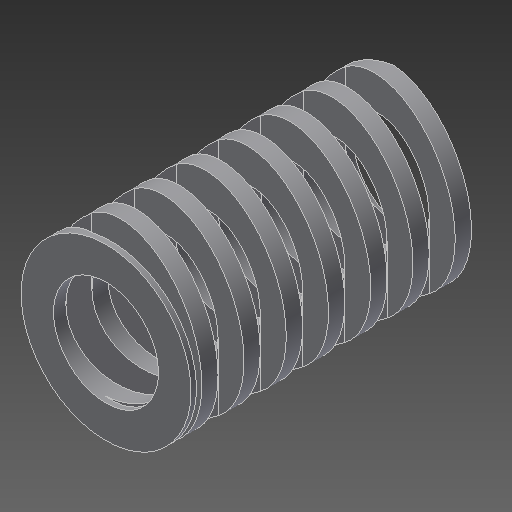
# Autodesk Inventor part: SWU17-30
Saved by Autodesk Inventor 2021.1 (Build 251245010, 245A)
## iProperties
Created: 2010-03-11
Part Number: SWU17-30
Catalog Web Link: www.cadenas.de
Document SubType Name: Modeling
Density: 1 g/cm^3
Material: MISUMI
Appearance: 既定
Category: PARTsolutions
NB: SWU17-30
NN: SWU
NT: Coil Springs - Super High Deflection - SWU
NBSYN: $PN.
LINA: SWU17-30
PN: SWU17-30
TYPE: SWU
MAT: Alloy Steel
D: 17.0
DD: 10.5
L: 30
L1: 20,25,30,35,40,45,50,55,60,65,70,75,80,90,100,110,120,125,150,175
LO: 8.17 {0.83}
LL: 9.00
F: 18.0
LO1: 147.1 {15.0}
X: 3.250
D1: 1.625
H1: 4.224
ANGLE: 5.000
KT: DUMMY
PSOL_IDENT_0: {\\10.0.0.149\dplatte\cadenas\23d-libs\misumi\metric\29_springs\swu.prj},156 {VTYP=3D},{NB=SWU17-30}
PSOL_IDENT_1: ,{LINA=SWU17-30},{NN=SWU},{DATE=18.02.2010 11:50:29},{GEOMDATE=18.02.2010 11:50:00},{VERSION=},{LINE
PSOL_IDENT_2: ID=40},{LINESUBID=-1},{WBVAR=L}  {NB=SWU17-30},{LINA=SWU17-30},{KT=DUMMY},{PN=SWU17-30},{TYPE=SWU},{
PSOL_IDENT_3: MAT=Alloy Steel},{D=17.0},{DD=10.5},{L=30},{L1=20,25,30,35,40,45,50,55,60,65,70,75,80,90,100,110,120
PSOL_IDENT_4: ,125,150,175},{LO=8.17 \{0.83\}},{LL=9.00},{F=18.0},{LO1=147.1 \{15.0\}},{X=3.25},{D1=1.625},{H1=4.2
PSOL_IDENT_5: 24},{ANGLE=5.000}
Title: コイルスプリング
Comments: Coil Springs - Super High Deflection - SWU
Autodesk Inventor part; units mm, degrees
ref_plane "YZ Plane" through (0, 0, 0) normal (1, 0, 0) x (0, 1, 0)
ref_plane "XZ Plane" through (0, 0, 0) normal (0, 1, 0) x (-1, 0, 0)
ref_plane "XY Plane" through (0, 0, 0) normal (0, 0, 1) x (1, 0, 0)
sketch "Sketch_1" plane through (0, 0, 0) normal (0, 0, 1) x (1, 0, 0)
  circle A0 centre (0, 0) radius 8.5
  circle A1 centre (0, 0) radius 5.25
  constraints: 2 centre point
extrude "Extrusion1" add sketch "Sketch_1" along normal blind 30
sketch "Sketch_2" plane through (0, 0, 0) normal (0, 1, 0) x (-1, 0, 0)
  line L0 (70.217, 56.4456) -> (8.5, 216.2365)
  line L1 (8.5, 216.2365) -> (8.5, 215.2652)
  line L2 (8.5, 215.2652) -> (5.25, 214.6115)
  line L3 (5.25, 214.6115) -> (-8.5, 217.3772)
  line L4 (-8.5, 217.3772) -> (-8.5, 214.7782)
  line L5 (-8.5, 214.7782) -> (5.25, 212.0125)
  line L6 (5.25, 212.0125) -> (8.5, 212.6662)
  line L7 (8.5, 212.6662) -> (8.5, 211.0412)
  line L8 (8.5, 211.0412) -> (5.25, 210.3875)
  line L9 (5.25, 210.3875) -> (-8.5, 213.1532)
  line L10 (-8.5, 213.1532) -> (-8.5, 210.5542)
  line L11 (-8.5, 210.5542) -> (5.25, 207.7885)
  line L12 (5.25, 207.7885) -> (8.5, 208.4422)
  line L13 (8.5, 208.4422) -> (8.5, 206.8172)
  line L14 (8.5, 206.8172) -> (5.25, 206.1635)
  line L15 (5.25, 206.1635) -> (-8.5, 208.9292)
  line L16 (-8.5, 208.9292) -> (-8.5, 206.3302)
  line L17 (-8.5, 206.3302) -> (5.25, 203.5645)
  line L18 (5.25, 203.5645) -> (8.5, 204.2182)
  line L19 (8.5, 204.2182) -> (8.5, 202.5932)
  line L20 (8.5, 202.5932) -> (5.25, 201.9395)
  line L21 (5.25, 201.9395) -> (-8.5, 204.7052)
  line L22 (-8.5, 204.7052) -> (-8.5, 202.1062)
  line L23 (-8.5, 202.1062) -> (5.25, 199.3405)
  line L24 (5.25, 199.3405) -> (8.5, 199.9942)
  line L25 (8.5, 199.9942) -> (8.5, 198.3692)
  line L26 (8.5, 198.3692) -> (5.25, 197.7155)
  line L27 (5.25, 197.7155) -> (-8.5, 200.4812)
  line L28 (-8.5, 200.4812) -> (-8.5, 197.8822)
  line L29 (-8.5, 197.8822) -> (5.25, 195.1165)
  line L30 (5.25, 195.1165) -> (8.5, 195.7702)
  line L31 (8.5, 195.7702) -> (8.5, 194.1452)
  line L32 (8.5, 194.1452) -> (5.25, 193.4915)
  line L33 (5.25, 193.4915) -> (-8.5, 196.2572)
  line L34 (-8.5, 196.2572) -> (-8.5, 193.6582)
  line L35 (-8.5, 193.6582) -> (5.25, 190.8925)
  line L36 (5.25, 190.8925) -> (8.5, 191.5462)
  line L37 (8.5, 191.5462) -> (8.5, 189.9212)
  line L38 (8.5, 189.9212) -> (5.25, 189.2675)
  line L39 (5.25, 189.2675) -> (-8.5, 192.0332)
  line L40 (-8.5, 192.0332) -> (-8.5, 189.4342)
  line L41 (-8.5, 189.4342) -> (5.25, 186.6685)
  line L42 (5.25, 186.6685) -> (8.5, 187.3222)
  line L43 (8.5, 187.3222) -> (8.5, 185.6972)
  line L44 (8.5, 185.6972) -> (5.25, 185.0435)
  line L45 (5.25, 185.0435) -> (-8.5, 187.8092)
  line L46 (-8.5, 187.8092) -> (-8.5, 185.2102)
  line L47 (-8.5, 185.2102) -> (5.25, 182.4445)
  line L48 (5.25, 182.4445) -> (8.5, 183.0982)
  line L49 (8.5, 183.0982) -> (8.5, 181.4732)
  line L50 (8.5, 181.4732) -> (5.25, 180.8195)
  line L51 (5.25, 180.8195) -> (-8.5, 183.5852)
  line L52 (-8.5, 183.5852) -> (-8.5, 180.9862)
  line L53 (-8.5, 180.9862) -> (5.25, 178.2205)
  line L54 (5.25, 178.2205) -> (8.5, 178.8742)
  line L55 (8.5, 178.8742) -> (8.5, 177.2492)
  line L56 (8.5, 177.2492) -> (5.25, 176.5955)
  line L57 (5.25, 176.5955) -> (-8.5, 179.3612)
  line L58 (-8.5, 179.3612) -> (-8.5, 176.7622)
  line L59 (-8.5, 176.7622) -> (5.25, 173.9965)
  line L60 (5.25, 173.9965) -> (8.5, 174.6502)
  line L61 (8.5, 174.6502) -> (8.5, 173.0252)
  line L62 (8.5, 173.0252) -> (5.25, 172.3715)
  line L63 (5.25, 172.3715) -> (-8.5, 175.1372)
  line L64 (-8.5, 175.1372) -> (-8.5, 172.5382)
  line L65 (-8.5, 172.5382) -> (5.25, 169.7725)
  line L66 (5.25, 169.7725) -> (8.5, 170.4262)
  line L67 (8.5, 170.4262) -> (8.5, 168.8012)
  line L68 (8.5, 168.8012) -> (5.25, 168.1475)
  line L69 (5.25, 168.1475) -> (-8.5, 170.9132)
  line L70 (-8.5, 170.9132) -> (-8.5, 168.3142)
  line L71 (-8.5, 168.3142) -> (5.25, 165.5485)
  line L72 (5.25, 165.5485) -> (8.5, 166.2022)
  line L73 (8.5, 166.2022) -> (8.5, 164.5772)
  line L74 (8.5, 164.5772) -> (5.25, 163.9235)
  line L75 (5.25, 163.9235) -> (-8.5, 166.6892)
  line L76 (-8.5, 166.6892) -> (-8.5, 164.0902)
  line L77 (-8.5, 164.0902) -> (5.25, 161.3245)
  line L78 (5.25, 161.3245) -> (8.5, 161.9782)
  line L79 (8.5, 161.9782) -> (8.5, 160.3532)
  line L80 (8.5, 160.3532) -> (5.25, 159.6995)
  line L81 (5.25, 159.6995) -> (-8.5, 162.4652)
  line L82 (-8.5, 162.4652) -> (-8.5, 159.8662)
  line L83 (-8.5, 159.8662) -> (5.25, 157.1005)
  line L84 (5.25, 157.1005) -> (8.5, 157.7542)
  line L85 (8.5, 157.7542) -> (8.5, 156.1292)
  line L86 (8.5, 156.1292) -> (5.25, 155.4755)
  line L87 (5.25, 155.4755) -> (-8.5, 158.2412)
  line L88 (-8.5, 158.2412) -> (-8.5, 155.6422)
  line L89 (-8.5, 155.6422) -> (5.25, 152.8765)
  line L90 (5.25, 152.8765) -> (8.5, 153.5302)
  line L91 (8.5, 153.5302) -> (8.5, 151.9052)
  line L92 (8.5, 151.9052) -> (5.25, 151.2515)
  line L93 (5.25, 151.2515) -> (-8.5, 154.0172)
  line L94 (-8.5, 154.0172) -> (-8.5, 151.4182)
  line L95 (-8.5, 151.4182) -> (5.25, 148.6525)
  line L96 (5.25, 148.6525) -> (8.5, 149.3062)
  line L97 (8.5, 149.3062) -> (8.5, 147.6812)
  line L98 (8.5, 147.6812) -> (5.25, 147.0275)
  line L99 (5.25, 147.0275) -> (-8.5, 149.7932)
  line L100 (-8.5, 149.7932) -> (-8.5, 147.1942)
  line L101 (-8.5, 147.1942) -> (5.25, 144.4285)
  line L102 (5.25, 144.4285) -> (8.5, 145.0822)
  line L103 (8.5, 145.0822) -> (8.5, 143.4572)
  line L104 (8.5, 143.4572) -> (5.25, 142.8035)
  line L105 (5.25, 142.8035) -> (-8.5, 145.5692)
  line L106 (-8.5, 145.5692) -> (-8.5, 142.9702)
  line L107 (-8.5, 142.9702) -> (5.25, 140.2045)
  line L108 (5.25, 140.2045) -> (8.5, 140.8582)
  line L109 (8.5, 140.8582) -> (8.5, 139.2332)
  line L110 (8.5, 139.2332) -> (5.25, 138.5795)
  line L111 (5.25, 138.5795) -> (-8.5, 141.3452)
  line L112 (-8.5, 141.3452) -> (-8.5, 138.7462)
  line L113 (-8.5, 138.7462) -> (5.25, 135.9805)
  line L114 (5.25, 135.9805) -> (8.5, 136.6342)
  line L115 (8.5, 136.6342) -> (8.5, 135.0092)
  line L116 (8.5, 135.0092) -> (5.25, 134.3555)
  line L117 (5.25, 134.3555) -> (-8.5, 137.1212)
  line L118 (-8.5, 137.1212) -> (-8.5, 134.5222)
  line L119 (-8.5, 134.5222) -> (5.25, 131.7565)
  line L120 (5.25, 131.7565) -> (8.5, 132.4102)
  line L121 (8.5, 132.4102) -> (8.5, 130.7852)
  line L122 (8.5, 130.7852) -> (5.25, 130.1315)
  line L123 (5.25, 130.1315) -> (-8.5, 132.8972)
  line L124 (-8.5, 132.8972) -> (-8.5, 130.2982)
  line L125 (-8.5, 130.2982) -> (5.25, 127.5325)
  line L126 (5.25, 127.5325) -> (8.5, 128.1862)
  line L127 (8.5, 128.1862) -> (8.5, 126.5612)
  line L128 (8.5, 126.5612) -> (5.25, 125.9075)
  line L129 (5.25, 125.9075) -> (-8.5, 128.6732)
  line L130 (-8.5, 128.6732) -> (-8.5, 126.0742)
  line L131 (-8.5, 126.0742) -> (5.25, 123.3085)
  line L132 (5.25, 123.3085) -> (8.5, 123.9622)
  line L133 (8.5, 123.9622) -> (8.5, 122.3372)
  line L134 (8.5, 122.3372) -> (5.25, 121.6835)
  line L135 (5.25, 121.6835) -> (-8.5, 124.4492)
  line L136 (-8.5, 124.4492) -> (-8.5, 121.8502)
  line L137 (-8.5, 121.8502) -> (5.25, 119.0845)
  line L138 (5.25, 119.0845) -> (8.5, 119.7382)
  line L139 (8.5, 119.7382) -> (8.5, 118.1132)
  line L140 (8.5, 118.1132) -> (5.25, 117.4595)
  line L141 (5.25, 117.4595) -> (-8.5, 120.2252)
  line L142 (-8.5, 120.2252) -> (-8.5, 117.6262)
  line L143 (-8.5, 117.6262) -> (5.25, 114.8605)
  line L144 (5.25, 114.8605) -> (8.5, 115.5142)
  line L145 (8.5, 115.5142) -> (8.5, 113.8892)
  line L146 (8.5, 113.8892) -> (5.25, 113.2355)
  line L147 (5.25, 113.2355) -> (-8.5, 116.0012)
  line L148 (-8.5, 116.0012) -> (-8.5, 113.4022)
  line L149 (-8.5, 113.4022) -> (5.25, 110.6365)
  line L150 (5.25, 110.6365) -> (8.5, 111.2902)
  line L151 (8.5, 111.2902) -> (8.5, 109.6652)
  line L152 (8.5, 109.6652) -> (5.25, 109.0115)
  line L153 (5.25, 109.0115) -> (-8.5, 111.7772)
  line L154 (-8.5, 111.7772) -> (-8.5, 109.1782)
  line L155 (-8.5, 109.1782) -> (5.25, 106.4125)
  line L156 (5.25, 106.4125) -> (8.5, 107.0662)
  line L157 (8.5, 107.0662) -> (8.5, 105.4412)
  line L158 (8.5, 105.4412) -> (5.25, 104.7875)
  line L159 (5.25, 104.7875) -> (-8.5, 107.5532)
  line L160 (-8.5, 107.5532) -> (-8.5, 104.9542)
  line L161 (-8.5, 104.9542) -> (5.25, 102.1885)
  line L162 (5.25, 102.1885) -> (8.5, 102.8422)
  line L163 (8.5, 102.8422) -> (8.5, 101.2172)
  line L164 (8.5, 101.2172) -> (5.25, 100.5635)
  line L165 (5.25, 100.5635) -> (-8.5, 103.3292)
  line L166 (-8.5, 103.3292) -> (-8.5, 100.7302)
  line L167 (-8.5, 100.7302) -> (5.25, 97.9645)
  line L168 (5.25, 97.9645) -> (8.5, 98.6182)
  line L169 (8.5, 98.6182) -> (8.5, 96.9932)
  line L170 (8.5, 96.9932) -> (5.25, 96.3395)
  line L171 (5.25, 96.3395) -> (-8.5, 99.1052)
  line L172 (-8.5, 99.1052) -> (-8.5, 96.5062)
  line L173 (-8.5, 96.5062) -> (5.25, 93.7405)
  line L174 (5.25, 93.7405) -> (8.5, 94.3942)
  line L175 (8.5, 94.3942) -> (8.5, 92.7692)
  line L176 (8.5, 92.7692) -> (5.25, 92.1155)
  line L177 (5.25, 92.1155) -> (-8.5, 94.8812)
  line L178 (-8.5, 94.8812) -> (-8.5, 92.2822)
  line L179 (-8.5, 92.2822) -> (5.25, 89.5165)
  line L180 (5.25, 89.5165) -> (8.5, 90.1702)
  line L181 (8.5, 90.1702) -> (8.5, 88.5452)
  line L182 (8.5, 88.5452) -> (5.25, 87.8915)
  line L183 (5.25, 87.8915) -> (-8.5, 90.6572)
  line L184 (-8.5, 90.6572) -> (-8.5, 88.0582)
  line L185 (-8.5, 88.0582) -> (5.25, 85.2925)
  line L186 (5.25, 85.2925) -> (8.5, 85.9462)
  line L187 (8.5, 85.9462) -> (8.5, 84.3212)
  line L188 (8.5, 84.3212) -> (5.25, 83.6675)
  line L189 (5.25, 83.6675) -> (-8.5, 86.4332)
  line L190 (-8.5, 86.4332) -> (-8.5, 83.8342)
  line L191 (-8.5, 83.8342) -> (5.25, 81.0685)
  line L192 (5.25, 81.0685) -> (8.5, 81.7222)
  line L193 (8.5, 81.7222) -> (8.5, 80.0972)
  line L194 (8.5, 80.0972) -> (5.25, 79.4435)
  line L195 (5.25, 79.4435) -> (-8.5, 82.2092)
  line L196 (-8.5, 82.2092) -> (-8.5, 79.6102)
  line L197 (-8.5, 79.6102) -> (5.25, 76.8445)
  line L198 (5.25, 76.8445) -> (8.5, 77.4982)
  line L199 (8.5, 77.4982) -> (8.5, 75.8732)
  line L200 (8.5, 75.8732) -> (5.25, 75.2195)
  line L201 (5.25, 75.2195) -> (-8.5, 77.9852)
  line L202 (-8.5, 77.9852) -> (-8.5, 75.3862)
  line L203 (-8.5, 75.3862) -> (5.25, 72.6205)
  line L204 (5.25, 72.6205) -> (8.5, 73.2742)
  line L205 (8.5, 73.2742) -> (8.5, 71.6492)
  line L206 (8.5, 71.6492) -> (5.25, 70.9955)
  line L207 (5.25, 70.9955) -> (-8.5, 73.7612)
  line L208 (-8.5, 73.7612) -> (-8.5, 71.1622)
  line L209 (-8.5, 71.1622) -> (5.25, 68.3965)
  line L210 (5.25, 68.3965) -> (8.5, 69.0502)
  line L211 (8.5, 69.0502) -> (8.5, 67.4252)
  line L212 (8.5, 67.4252) -> (5.25, 66.7715)
  line L213 (5.25, 66.7715) -> (-8.5, 69.5372)
  line L214 (-8.5, 69.5372) -> (-8.5, 66.9382)
  line L215 (-8.5, 66.9382) -> (5.25, 64.1725)
  line L216 (5.25, 64.1725) -> (8.5, 64.8262)
  line L217 (8.5, 64.8262) -> (8.5, 63.2012)
  line L218 (8.5, 63.2012) -> (5.25, 62.5475)
  line L219 (5.25, 62.5475) -> (-8.5, 65.3132)
  line L220 (-8.5, 65.3132) -> (-8.5, 62.7142)
  line L221 (-8.5, 62.7142) -> (5.25, 59.9485)
  line L222 (5.25, 59.9485) -> (8.5, 60.6022)
  line L223 (8.5, 60.6022) -> (8.5, 58.9772)
  line L224 (8.5, 58.9772) -> (5.25, 58.3235)
  line L225 (5.25, 58.3235) -> (-8.5, 61.0892)
  line L226 (-8.5, 61.0892) -> (-8.5, 58.4902)
  line L227 (-8.5, 58.4902) -> (5.25, 55.7245)
  line L228 (5.25, 55.7245) -> (8.5, 56.3782)
  line L229 (8.5, 56.3782) -> (8.5, 54.7532)
  line L230 (8.5, 54.7532) -> (5.25, 54.0995)
  line L231 (5.25, 54.0995) -> (-8.5, 56.8652)
  line L232 (-8.5, 56.8652) -> (-8.5, 54.2662)
  line L233 (-8.5, 54.2662) -> (5.25, 51.5005)
  line L234 (5.25, 51.5005) -> (8.5, 52.1542)
  line L235 (8.5, 52.1542) -> (8.5, 50.5292)
  line L236 (8.5, 50.5292) -> (5.25, 49.8755)
  line L237 (5.25, 49.8755) -> (-8.5, 52.6412)
  line L238 (-8.5, 52.6412) -> (-8.5, 50.0422)
  line L239 (-8.5, 50.0422) -> (5.25, 47.2765)
  line L240 (5.25, 47.2765) -> (8.5, 47.9302)
  line L241 (8.5, 47.9302) -> (8.5, 46.3052)
  line L242 (8.5, 46.3052) -> (5.25, 45.6515)
  line L243 (5.25, 45.6515) -> (-8.5, 48.4172)
  line L244 (-8.5, 48.4172) -> (-8.5, 45.8182)
  line L245 (-8.5, 45.8182) -> (5.25, 43.0525)
  line L246 (5.25, 43.0525) -> (8.5, 43.7062)
  line L247 (8.5, 43.7062) -> (8.5, 42.0812)
  line L248 (8.5, 42.0812) -> (5.25, 41.4275)
  line L249 (5.25, 41.4275) -> (-8.5, 44.1932)
  line L250 (-8.5, 44.1932) -> (-8.5, 41.5942)
  line L251 (-8.5, 41.5942) -> (5.25, 38.8285)
  line L252 (5.25, 38.8285) -> (8.5, 39.4822)
  line L253 (8.5, 39.4822) -> (8.5, 37.8572)
  line L254 (8.5, 37.8572) -> (5.25, 37.2035)
  line L255 (5.25, 37.2035) -> (-8.5, 39.9692)
  line L256 (-8.5, 39.9692) -> (-8.5, 37.3702)
  line L257 (-8.5, 37.3702) -> (5.25, 34.6045)
  line L258 (5.25, 34.6045) -> (8.5, 35.2582)
  line L259 (8.5, 35.2582) -> (8.5, 33.6332)
  line L260 (8.5, 33.6332) -> (5.25, 32.9795)
  line L261 (5.25, 32.9795) -> (-8.5, 35.7452)
  line L262 (-8.5, 35.7452) -> (-8.5, 33.1462)
  line L263 (-8.5, 33.1462) -> (5.25, 30.3805)
  line L264 (5.25, 30.3805) -> (8.5, 31.0342)
  line L265 (8.5, 31.0342) -> (8.5, 29.4092)
  line L266 (8.5, 29.4092) -> (5.25, 28.7555)
  line L267 (5.25, 28.7555) -> (-8.5, 31.5212)
  line L268 (-8.5, 31.5212) -> (-8.5, 28.9222)
  line L269 (-8.5, 28.9222) -> (5.25, 26.1565)
  line L270 (5.25, 26.1565) -> (8.5, 26.8102)
  line L271 (8.5, 26.8102) -> (8.5, 25.1852)
  line L272 (8.5, 25.1852) -> (5.25, 24.5315)
  line L273 (5.25, 24.5315) -> (-8.5, 27.2972)
  line L274 (-8.5, 27.2972) -> (-8.5, 24.6982)
  line L275 (-8.5, 24.6982) -> (5.25, 21.9325)
  line L276 (5.25, 21.9325) -> (8.5, 22.5862)
  line L277 (8.5, 22.5862) -> (8.5, 20.9612)
  line L278 (8.5, 20.9612) -> (5.25, 20.3075)
  line L279 (5.25, 20.3075) -> (-8.5, 23.0732)
  line L280 (-8.5, 23.0732) -> (-8.5, 20.4742)
  line L281 (-8.5, 20.4742) -> (5.25, 17.7085)
  line L282 (5.25, 17.7085) -> (8.5, 18.3622)
  line L283 (8.5, 18.3622) -> (8.5, 16.7372)
  line L284 (8.5, 16.7372) -> (5.25, 16.0835)
  line L285 (5.25, 16.0835) -> (-8.5, 18.8492)
  line L286 (-8.5, 18.8492) -> (-8.5, 16.2502)
  line L287 (-8.5, 16.2502) -> (5.25, 13.4845)
  line L288 (5.25, 13.4845) -> (8.5, 14.1382)
  line L289 (8.5, 14.1382) -> (8.5, 12.5132)
  line L290 (8.5, 12.5132) -> (5.25, 11.8595)
  line L291 (5.25, 11.8595) -> (-8.5, 14.6252)
  line L292 (-8.5, 14.6252) -> (-8.5, 12.0262)
  line L293 (-8.5, 12.0262) -> (5.25, 9.2605)
  line L294 (5.25, 9.2605) -> (8.5, 9.9142)
  line L295 (8.5, 9.9142) -> (8.5, 8.2892)
  line L296 (8.5, 8.2892) -> (5.25, 7.6355)
  line L297 (5.25, 7.6355) -> (-8.5, 10.4012)
  line L298 (-8.5, 10.4012) -> (-8.5, 7.8022)
  line L299 (-8.5, 7.8022) -> (5.25, 5.0365)
  line L300 (5.25, 5.0365) -> (8.5, 5.6902)
  line L301 (8.5, 5.6902) -> (8.5, 4.0652)
  line L302 (8.5, 4.0652) -> (5.25, 3.4115)
  line L303 (5.25, 3.4115) -> (-8.5, 6.1772)
  line L304 (-8.5, 6.1772) -> (-8.5, 3.5782)
  line L305 (-8.5, 3.5782) -> (5.25, 0.8125)
  line L306 (5.25, 0.8125) -> (8.5, 1.4662)
  line L307 (8.5, 1.4662) -> (8.5, -0.1588)
  line L308 (8.5, -0.1588) -> (5.25, -0.8125)
  line L309 (5.25, -0.8125) -> (-8.5, 1.9532)
  line L310 (-8.5, 1.9532) -> (-8.5, -0.6458)
  line L311 (-8.5, -0.6458) -> (5.25, -3.4115)
  line L312 (5.25, -3.4115) -> (8.5, -2.7578)
  line L313 (8.5, -2.7578) -> (8.5, -3.4115)
  line L314 (8.5, -3.4115) -> (70.217, 56.4456)
  constraints: 630 end point
extrude "Extrusion2" cut sketch "Sketch_2" along normal blind 30
sketch "Sketch_3" plane through (0, 0, 0) normal (0, 1, 0) x (-1, 0, 0)
  line L0 (8.5, 5.6902) -> (8.5, 8.2892)
  line L1 (8.5, 8.2892) -> (-5.25, 5.5235)
  line L2 (-5.25, 5.5235) -> (-8.5, 6.1772)
  line L3 (-8.5, 6.1772) -> (-8.5, 7.8022)
  line L4 (-8.5, 7.8022) -> (-5.25, 7.1485)
  line L5 (-5.25, 7.1485) -> (8.5, 9.9142)
  line L6 (8.5, 9.9142) -> (8.5, 12.5132)
  line L7 (8.5, 12.5132) -> (-5.25, 9.7475)
  line L8 (-5.25, 9.7475) -> (-8.5, 10.4012)
  line L9 (-8.5, 10.4012) -> (-8.5, 12.0262)
  line L10 (-8.5, 12.0262) -> (-5.25, 11.3725)
  line L11 (-5.25, 11.3725) -> (8.5, 14.1382)
  line L12 (8.5, 14.1382) -> (8.5, 16.7372)
  line L13 (8.5, 16.7372) -> (-5.25, 13.9715)
  line L14 (-5.25, 13.9715) -> (-8.5, 14.6252)
  line L15 (-8.5, 14.6252) -> (-8.5, 16.2502)
  line L16 (-8.5, 16.2502) -> (-5.25, 15.5965)
  line L17 (-5.25, 15.5965) -> (8.5, 18.3622)
  line L18 (8.5, 18.3622) -> (8.5, 20.9612)
  line L19 (8.5, 20.9612) -> (-5.25, 18.1955)
  line L20 (-5.25, 18.1955) -> (-8.5, 18.8492)
  line L21 (-8.5, 18.8492) -> (-8.5, 20.4742)
  line L22 (-8.5, 20.4742) -> (-5.25, 19.8205)
  line L23 (-5.25, 19.8205) -> (8.5, 22.5862)
  line L24 (8.5, 22.5862) -> (8.5, 25.1852)
  line L25 (8.5, 25.1852) -> (-5.25, 22.4195)
  line L26 (-5.25, 22.4195) -> (-8.5, 23.0732)
  line L27 (-8.5, 23.0732) -> (-8.5, 24.6982)
  line L28 (-8.5, 24.6982) -> (-5.25, 24.0445)
  line L29 (-5.25, 24.0445) -> (8.5, 26.8102)
  line L30 (8.5, 26.8102) -> (8.5, 29.4092)
  line L31 (8.5, 29.4092) -> (-5.25, 26.6435)
  line L32 (-5.25, 26.6435) -> (-8.5, 27.2972)
  line L33 (-8.5, 27.2972) -> (-8.5, 28.9222)
  line L34 (-8.5, 28.9222) -> (-5.25, 28.2685)
  line L35 (-5.25, 28.2685) -> (8.5, 31.0342)
  line L36 (8.5, 31.0342) -> (8.5, 33.6332)
  line L37 (8.5, 33.6332) -> (-5.25, 30.8675)
  line L38 (-5.25, 30.8675) -> (-8.5, 31.5212)
  line L39 (-8.5, 31.5212) -> (-8.5, 33.1462)
  line L40 (-8.5, 33.1462) -> (-5.25, 32.4925)
  line L41 (-5.25, 32.4925) -> (8.5, 35.2582)
  line L42 (8.5, 35.2582) -> (8.5, 37.8572)
  line L43 (8.5, 37.8572) -> (-5.25, 35.0915)
  line L44 (-5.25, 35.0915) -> (-8.5, 35.7452)
  line L45 (-8.5, 35.7452) -> (-8.5, 37.3702)
  line L46 (-8.5, 37.3702) -> (-5.25, 36.7165)
  line L47 (-5.25, 36.7165) -> (8.5, 39.4822)
  line L48 (8.5, 39.4822) -> (8.5, 42.0812)
  line L49 (8.5, 42.0812) -> (-5.25, 39.3155)
  line L50 (-5.25, 39.3155) -> (-8.5, 39.9692)
  line L51 (-8.5, 39.9692) -> (-8.5, 41.5942)
  line L52 (-8.5, 41.5942) -> (-5.25, 40.9405)
  line L53 (-5.25, 40.9405) -> (8.5, 43.7062)
  line L54 (8.5, 43.7062) -> (8.5, 46.3052)
  line L55 (8.5, 46.3052) -> (-5.25, 43.5395)
  line L56 (-5.25, 43.5395) -> (-8.5, 44.1932)
  line L57 (-8.5, 44.1932) -> (-8.5, 45.8182)
  line L58 (-8.5, 45.8182) -> (-5.25, 45.1645)
  line L59 (-5.25, 45.1645) -> (8.5, 47.9302)
  line L60 (8.5, 47.9302) -> (8.5, 50.5292)
  line L61 (8.5, 50.5292) -> (-5.25, 47.7635)
  line L62 (-5.25, 47.7635) -> (-8.5, 48.4172)
  line L63 (-8.5, 48.4172) -> (-8.5, 50.0422)
  line L64 (-8.5, 50.0422) -> (-5.25, 49.3885)
  line L65 (-5.25, 49.3885) -> (8.5, 52.1542)
  line L66 (8.5, 52.1542) -> (8.5, 54.7532)
  line L67 (8.5, 54.7532) -> (-5.25, 51.9875)
  line L68 (-5.25, 51.9875) -> (-8.5, 52.6412)
  line L69 (-8.5, 52.6412) -> (-8.5, 54.2662)
  line L70 (-8.5, 54.2662) -> (-5.25, 53.6125)
  line L71 (-5.25, 53.6125) -> (8.5, 56.3782)
  line L72 (8.5, 56.3782) -> (8.5, 58.9772)
  line L73 (8.5, 58.9772) -> (-5.25, 56.2115)
  line L74 (-5.25, 56.2115) -> (-8.5, 56.8652)
  line L75 (-8.5, 56.8652) -> (-8.5, 58.4902)
  line L76 (-8.5, 58.4902) -> (-5.25, 57.8365)
  line L77 (-5.25, 57.8365) -> (8.5, 60.6022)
  line L78 (8.5, 60.6022) -> (8.5, 63.2012)
  line L79 (8.5, 63.2012) -> (-5.25, 60.4355)
  line L80 (-5.25, 60.4355) -> (-8.5, 61.0892)
  line L81 (-8.5, 61.0892) -> (-8.5, 62.7142)
  line L82 (-8.5, 62.7142) -> (-5.25, 62.0605)
  line L83 (-5.25, 62.0605) -> (8.5, 64.8262)
  line L84 (8.5, 64.8262) -> (8.5, 67.4252)
  line L85 (8.5, 67.4252) -> (-5.25, 64.6595)
  line L86 (-5.25, 64.6595) -> (-8.5, 65.3132)
  line L87 (-8.5, 65.3132) -> (-8.5, 66.9382)
  line L88 (-8.5, 66.9382) -> (-5.25, 66.2845)
  line L89 (-5.25, 66.2845) -> (8.5, 69.0502)
  line L90 (8.5, 69.0502) -> (8.5, 71.6492)
  line L91 (8.5, 71.6492) -> (-5.25, 68.8835)
  line L92 (-5.25, 68.8835) -> (-8.5, 69.5372)
  line L93 (-8.5, 69.5372) -> (-8.5, 71.1622)
  line L94 (-8.5, 71.1622) -> (-5.25, 70.5085)
  line L95 (-5.25, 70.5085) -> (8.5, 73.2742)
  line L96 (8.5, 73.2742) -> (8.5, 75.8732)
  line L97 (8.5, 75.8732) -> (-5.25, 73.1075)
  line L98 (-5.25, 73.1075) -> (-8.5, 73.7612)
  line L99 (-8.5, 73.7612) -> (-8.5, 75.3862)
  line L100 (-8.5, 75.3862) -> (-5.25, 74.7325)
  line L101 (-5.25, 74.7325) -> (8.5, 77.4982)
  line L102 (8.5, 77.4982) -> (8.5, 80.0972)
  line L103 (8.5, 80.0972) -> (-5.25, 77.3315)
  line L104 (-5.25, 77.3315) -> (-8.5, 77.9852)
  line L105 (-8.5, 77.9852) -> (-8.5, 79.6102)
  line L106 (-8.5, 79.6102) -> (-5.25, 78.9565)
  line L107 (-5.25, 78.9565) -> (8.5, 81.7222)
  line L108 (8.5, 81.7222) -> (8.5, 84.3212)
  line L109 (8.5, 84.3212) -> (-5.25, 81.5555)
  line L110 (-5.25, 81.5555) -> (-8.5, 82.2092)
  line L111 (-8.5, 82.2092) -> (-8.5, 83.8342)
  line L112 (-8.5, 83.8342) -> (-5.25, 83.1805)
  line L113 (-5.25, 83.1805) -> (8.5, 85.9462)
  line L114 (8.5, 85.9462) -> (8.5, 88.5452)
  line L115 (8.5, 88.5452) -> (-5.25, 85.7795)
  line L116 (-5.25, 85.7795) -> (-8.5, 86.4332)
  line L117 (-8.5, 86.4332) -> (-8.5, 88.0582)
  line L118 (-8.5, 88.0582) -> (-5.25, 87.4045)
  line L119 (-5.25, 87.4045) -> (8.5, 90.1702)
  line L120 (8.5, 90.1702) -> (8.5, 92.7692)
  line L121 (8.5, 92.7692) -> (-5.25, 90.0035)
  line L122 (-5.25, 90.0035) -> (-8.5, 90.6572)
  line L123 (-8.5, 90.6572) -> (-8.5, 92.2822)
  line L124 (-8.5, 92.2822) -> (-5.25, 91.6285)
  line L125 (-5.25, 91.6285) -> (8.5, 94.3942)
  line L126 (8.5, 94.3942) -> (8.5, 96.9932)
  line L127 (8.5, 96.9932) -> (-5.25, 94.2275)
  line L128 (-5.25, 94.2275) -> (-8.5, 94.8812)
  line L129 (-8.5, 94.8812) -> (-8.5, 96.5062)
  line L130 (-8.5, 96.5062) -> (-5.25, 95.8525)
  line L131 (-5.25, 95.8525) -> (8.5, 98.6182)
  line L132 (8.5, 98.6182) -> (8.5, 101.2172)
  line L133 (8.5, 101.2172) -> (-5.25, 98.4515)
  line L134 (-5.25, 98.4515) -> (-8.5, 99.1052)
  line L135 (-8.5, 99.1052) -> (-8.5, 100.7302)
  line L136 (-8.5, 100.7302) -> (-5.25, 100.0765)
  line L137 (-5.25, 100.0765) -> (8.5, 102.8422)
  line L138 (8.5, 102.8422) -> (8.5, 105.4412)
  line L139 (8.5, 105.4412) -> (-5.25, 102.6755)
  line L140 (-5.25, 102.6755) -> (-8.5, 103.3292)
  line L141 (-8.5, 103.3292) -> (-8.5, 104.9542)
  line L142 (-8.5, 104.9542) -> (-5.25, 104.3005)
  line L143 (-5.25, 104.3005) -> (8.5, 107.0662)
  line L144 (8.5, 107.0662) -> (8.5, 109.6652)
  line L145 (8.5, 109.6652) -> (-5.25, 106.8995)
  line L146 (-5.25, 106.8995) -> (-8.5, 107.5532)
  line L147 (-8.5, 107.5532) -> (-8.5, 109.1782)
  line L148 (-8.5, 109.1782) -> (-5.25, 108.5245)
  line L149 (-5.25, 108.5245) -> (8.5, 111.2902)
  line L150 (8.5, 111.2902) -> (8.5, 113.8892)
  line L151 (8.5, 113.8892) -> (-5.25, 111.1235)
  line L152 (-5.25, 111.1235) -> (-8.5, 111.7772)
  line L153 (-8.5, 111.7772) -> (-8.5, 113.4022)
  line L154 (-8.5, 113.4022) -> (-5.25, 112.7485)
  line L155 (-5.25, 112.7485) -> (8.5, 115.5142)
  line L156 (8.5, 115.5142) -> (8.5, 118.1132)
  line L157 (8.5, 118.1132) -> (-5.25, 115.3475)
  line L158 (-5.25, 115.3475) -> (-8.5, 116.0012)
  line L159 (-8.5, 116.0012) -> (-8.5, 117.6262)
  line L160 (-8.5, 117.6262) -> (-5.25, 116.9725)
  line L161 (-5.25, 116.9725) -> (8.5, 119.7382)
  line L162 (8.5, 119.7382) -> (8.5, 122.3372)
  line L163 (8.5, 122.3372) -> (-5.25, 119.5715)
  line L164 (-5.25, 119.5715) -> (-8.5, 120.2252)
  line L165 (-8.5, 120.2252) -> (-8.5, 121.8502)
  line L166 (-8.5, 121.8502) -> (-5.25, 121.1965)
  line L167 (-5.25, 121.1965) -> (8.5, 123.9622)
  line L168 (8.5, 123.9622) -> (8.5, 126.5612)
  line L169 (8.5, 126.5612) -> (-5.25, 123.7955)
  line L170 (-5.25, 123.7955) -> (-8.5, 124.4492)
  line L171 (-8.5, 124.4492) -> (-8.5, 126.0742)
  line L172 (-8.5, 126.0742) -> (-5.25, 125.4205)
  line L173 (-5.25, 125.4205) -> (8.5, 128.1862)
  line L174 (8.5, 128.1862) -> (8.5, 130.7852)
  line L175 (8.5, 130.7852) -> (-5.25, 128.0195)
  line L176 (-5.25, 128.0195) -> (-8.5, 128.6732)
  line L177 (-8.5, 128.6732) -> (-8.5, 130.2982)
  line L178 (-8.5, 130.2982) -> (-5.25, 129.6445)
  line L179 (-5.25, 129.6445) -> (8.5, 132.4102)
  line L180 (8.5, 132.4102) -> (8.5, 135.0092)
  line L181 (8.5, 135.0092) -> (-5.25, 132.2435)
  line L182 (-5.25, 132.2435) -> (-8.5, 132.8972)
  line L183 (-8.5, 132.8972) -> (-8.5, 134.5222)
  line L184 (-8.5, 134.5222) -> (-5.25, 133.8685)
  line L185 (-5.25, 133.8685) -> (8.5, 136.6342)
  line L186 (8.5, 136.6342) -> (8.5, 139.2332)
  line L187 (8.5, 139.2332) -> (-5.25, 136.4675)
  line L188 (-5.25, 136.4675) -> (-8.5, 137.1212)
  line L189 (-8.5, 137.1212) -> (-8.5, 138.7462)
  line L190 (-8.5, 138.7462) -> (-5.25, 138.0925)
  line L191 (-5.25, 138.0925) -> (8.5, 140.8582)
  line L192 (8.5, 140.8582) -> (8.5, 143.4572)
  line L193 (8.5, 143.4572) -> (-5.25, 140.6915)
  line L194 (-5.25, 140.6915) -> (-8.5, 141.3452)
  line L195 (-8.5, 141.3452) -> (-8.5, 142.9702)
  line L196 (-8.5, 142.9702) -> (-5.25, 142.3165)
  line L197 (-5.25, 142.3165) -> (8.5, 145.0822)
  line L198 (8.5, 145.0822) -> (8.5, 147.6812)
  line L199 (8.5, 147.6812) -> (-5.25, 144.9155)
  line L200 (-5.25, 144.9155) -> (-8.5, 145.5692)
  line L201 (-8.5, 145.5692) -> (-8.5, 147.1942)
  line L202 (-8.5, 147.1942) -> (-5.25, 146.5405)
  line L203 (-5.25, 146.5405) -> (8.5, 149.3062)
  line L204 (8.5, 149.3062) -> (8.5, 151.9052)
  line L205 (8.5, 151.9052) -> (-5.25, 149.1395)
  line L206 (-5.25, 149.1395) -> (-8.5, 149.7932)
  line L207 (-8.5, 149.7932) -> (-8.5, 151.4182)
  line L208 (-8.5, 151.4182) -> (-5.25, 150.7645)
  line L209 (-5.25, 150.7645) -> (8.5, 153.5302)
  line L210 (8.5, 153.5302) -> (8.5, 156.1292)
  line L211 (8.5, 156.1292) -> (-5.25, 153.3635)
  line L212 (-5.25, 153.3635) -> (-8.5, 154.0172)
  line L213 (-8.5, 154.0172) -> (-8.5, 155.6422)
  line L214 (-8.5, 155.6422) -> (-5.25, 154.9885)
  line L215 (-5.25, 154.9885) -> (8.5, 157.7542)
  line L216 (8.5, 157.7542) -> (8.5, 160.3532)
  line L217 (8.5, 160.3532) -> (-5.25, 157.5875)
  line L218 (-5.25, 157.5875) -> (-8.5, 158.2412)
  line L219 (-8.5, 158.2412) -> (-8.5, 159.8662)
  line L220 (-8.5, 159.8662) -> (-5.25, 159.2125)
  line L221 (-5.25, 159.2125) -> (8.5, 161.9782)
  line L222 (8.5, 161.9782) -> (8.5, 164.5772)
  line L223 (8.5, 164.5772) -> (-5.25, 161.8115)
  line L224 (-5.25, 161.8115) -> (-8.5, 162.4652)
  line L225 (-8.5, 162.4652) -> (-8.5, 164.0902)
  line L226 (-8.5, 164.0902) -> (-5.25, 163.4365)
  line L227 (-5.25, 163.4365) -> (8.5, 166.2022)
  line L228 (8.5, 166.2022) -> (8.5, 168.8012)
  line L229 (8.5, 168.8012) -> (-5.25, 166.0355)
  line L230 (-5.25, 166.0355) -> (-8.5, 166.6892)
  line L231 (-8.5, 166.6892) -> (-8.5, 168.3142)
  line L232 (-8.5, 168.3142) -> (-5.25, 167.6605)
  line L233 (-5.25, 167.6605) -> (8.5, 170.4262)
  line L234 (8.5, 170.4262) -> (8.5, 173.0252)
  line L235 (8.5, 173.0252) -> (-5.25, 170.2595)
  line L236 (-5.25, 170.2595) -> (-8.5, 170.9132)
  line L237 (-8.5, 170.9132) -> (-8.5, 172.5382)
  line L238 (-8.5, 172.5382) -> (-5.25, 171.8845)
  line L239 (-5.25, 171.8845) -> (8.5, 174.6502)
  line L240 (8.5, 174.6502) -> (8.5, 177.2492)
  line L241 (8.5, 177.2492) -> (-5.25, 174.4835)
  line L242 (-5.25, 174.4835) -> (-8.5, 175.1372)
  line L243 (-8.5, 175.1372) -> (-8.5, 176.7622)
  line L244 (-8.5, 176.7622) -> (-5.25, 176.1085)
  line L245 (-5.25, 176.1085) -> (8.5, 178.8742)
  line L246 (8.5, 178.8742) -> (8.5, 181.4732)
  line L247 (8.5, 181.4732) -> (-5.25, 178.7075)
  line L248 (-5.25, 178.7075) -> (-8.5, 179.3612)
  line L249 (-8.5, 179.3612) -> (-8.5, 180.9862)
  line L250 (-8.5, 180.9862) -> (-5.25, 180.3325)
  line L251 (-5.25, 180.3325) -> (8.5, 183.0982)
  line L252 (8.5, 183.0982) -> (8.5, 185.6972)
  line L253 (8.5, 185.6972) -> (-5.25, 182.9315)
  line L254 (-5.25, 182.9315) -> (-8.5, 183.5852)
  line L255 (-8.5, 183.5852) -> (-8.5, 185.2102)
  line L256 (-8.5, 185.2102) -> (-5.25, 184.5565)
  line L257 (-5.25, 184.5565) -> (8.5, 187.3222)
  line L258 (8.5, 187.3222) -> (8.5, 189.9212)
  line L259 (8.5, 189.9212) -> (-5.25, 187.1555)
  line L260 (-5.25, 187.1555) -> (-8.5, 187.8092)
  line L261 (-8.5, 187.8092) -> (-8.5, 189.4342)
  line L262 (-8.5, 189.4342) -> (-5.25, 188.7805)
  line L263 (-5.25, 188.7805) -> (8.5, 191.5462)
  line L264 (8.5, 191.5462) -> (8.5, 194.1452)
  line L265 (8.5, 194.1452) -> (-5.25, 191.3795)
  line L266 (-5.25, 191.3795) -> (-8.5, 192.0332)
  line L267 (-8.5, 192.0332) -> (-8.5, 193.6582)
  line L268 (-8.5, 193.6582) -> (-5.25, 193.0045)
  line L269 (-5.25, 193.0045) -> (8.5, 195.7702)
  line L270 (8.5, 195.7702) -> (8.5, 198.3692)
  line L271 (8.5, 198.3692) -> (-5.25, 195.6035)
  line L272 (-5.25, 195.6035) -> (-8.5, 196.2572)
  line L273 (-8.5, 196.2572) -> (-8.5, 197.8822)
  line L274 (-8.5, 197.8822) -> (-5.25, 197.2285)
  line L275 (-5.25, 197.2285) -> (8.5, 199.9942)
  line L276 (8.5, 199.9942) -> (8.5, 202.5932)
  line L277 (8.5, 202.5932) -> (-5.25, 199.8275)
  line L278 (-5.25, 199.8275) -> (-8.5, 200.4812)
  line L279 (-8.5, 200.4812) -> (-8.5, 202.1062)
  line L280 (-8.5, 202.1062) -> (-5.25, 201.4525)
  line L281 (-5.25, 201.4525) -> (8.5, 204.2182)
  line L282 (8.5, 204.2182) -> (8.5, 206.8172)
  line L283 (8.5, 206.8172) -> (-5.25, 204.0515)
  line L284 (-5.25, 204.0515) -> (-8.5, 204.7052)
  line L285 (-8.5, 204.7052) -> (-8.5, 206.3302)
  line L286 (-8.5, 206.3302) -> (-5.25, 205.6765)
  line L287 (-5.25, 205.6765) -> (8.5, 208.4422)
  line L288 (8.5, 208.4422) -> (8.5, 211.0412)
  line L289 (8.5, 211.0412) -> (-5.25, 208.2755)
  line L290 (-5.25, 208.2755) -> (-8.5, 208.9292)
  line L291 (-8.5, 208.9292) -> (-8.5, 210.5542)
  line L292 (-8.5, 210.5542) -> (-5.25, 209.9005)
  line L293 (-5.25, 209.9005) -> (8.5, 212.6662)
  line L294 (8.5, 212.6662) -> (8.5, 215.2652)
  line L295 (8.5, 215.2652) -> (-5.25, 212.4995)
  line L296 (-5.25, 212.4995) -> (-8.5, 213.1532)
  line L297 (-8.5, 213.1532) -> (-8.5, 214.7782)
  line L298 (-8.5, 214.7782) -> (-5.25, 214.1245)
  line L299 (-5.25, 214.1245) -> (8.5, 216.8902)
  line L300 (8.5, 216.8902) -> (8.5, 219.4892)
  line L301 (8.5, 219.4892) -> (-5.25, 216.7235)
  line L302 (-5.25, 216.7235) -> (-8.5, 217.3772)
  line L303 (-8.5, 217.3772) -> (-8.5, 218.3485)
  line L304 (-8.5, 218.3485) -> (-62.1671, 62.3128)
  line L305 (-62.1671, 62.3128) -> (-8.5, -5.5235)
  line L306 (-8.5, -5.5235) -> (-8.5, -4.8698)
  line L307 (-8.5, -4.8698) -> (-5.25, -5.5235)
  line L308 (-5.25, -5.5235) -> (8.5, -2.7578)
  line L309 (8.5, -2.7578) -> (8.5, -0.1588)
  line L310 (8.5, -0.1588) -> (-5.25, -2.9245)
  line L311 (-5.25, -2.9245) -> (-8.5, -2.2708)
  line L312 (-8.5, -2.2708) -> (-8.5, -0.6458)
  line L313 (-8.5, -0.6458) -> (-5.25, -1.2995)
  line L314 (-5.25, -1.2995) -> (8.5, 1.4662)
  line L315 (8.5, 1.4662) -> (8.5, 4.0652)
  line L316 (8.5, 4.0652) -> (-5.25, 1.2995)
  line L317 (-5.25, 1.2995) -> (-8.5, 1.9532)
  line L318 (-8.5, 1.9532) -> (-8.5, 3.5782)
  line L319 (-8.5, 3.5782) -> (-5.25, 2.9245)
  line L320 (-5.25, 2.9245) -> (8.5, 5.6902)
  constraints: 642 end point
extrude "Extrusion3" cut sketch "Sketch_3" against normal blind 30
sketch "Sketch_4" plane through (0, 0, 30) normal (0, 0, 1) x (1, 0, 0)
  circle A0 centre (0, 0) radius 8.5
  circle A1 centre (0, 0) radius 5.25
  constraints: 2 centre point
extrude "Extrusion4" add sketch "Sketch_4" against normal blind 0.5417
